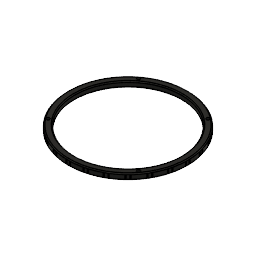
IR Ring v1 (Autodesk Fusion 360 design; units mm, degrees)
Autodesk Fusion 360 part; units mm, degrees
note: some values were not read from the file. Set by a fixed rule: which sketch regions a step uses.
sketch "Sketch1" plane through (0, 0, 0) normal (0, 1, 0) x (1, 0, 0)
  circle A0 centre (0, 0) radius 62 construction
  circle A1 centre (0, 0) radius 65
  circle A2 centre (0, 0) radius 58
  line L0 (0, 0) -> (-49.1879, -37.7432)
  line L1 (0, 0) -> (62, 0) construction
  line L2 (0, 0) -> (-37.7432, 49.1879)
  line L3 (0, 0) -> (0, -65) construction
  line L4 (0, 0) -> (49.1879, -37.7432)
  line L5 (0, 0) -> (37.7432, 49.1879)
  circle A3 centre (-49.1879, -37.7432) radius 1.65
  circle A4 centre (49.1879, -37.7432) radius 1.65
  circle A5 centre (37.7432, 49.1879) radius 1.65
  circle A6 centre (-37.7432, 49.1879) radius 1.65
  line L6 (0, 0) -> (0, 62) construction
  line L7 (3.4, 63.25) -> (-3.4, 63.25)
  line L8 (-3.4, 63.25) -> (-3.4, 60.75)
  line L9 (-3.4, 60.75) -> (3.4, 60.75)
  line L10 (3.4, 60.75) -> (3.4, 63.25)
  line L11 (3.4, 63.25) -> (-3.4, 60.75) construction
  line L12 (-3.4, 63.25) -> (3.4, 60.75) construction
  line L13 (3.6, 60.55) -> (-3.6, 60.55)
  line L14 (-3.6, 60.55) -> (-3.6, 63.45)
  line L15 (-3.6, 63.45) -> (3.6, 63.45)
  line L16 (3.6, 63.45) -> (3.6, 60.55)
  line L17 (3.6, 60.55) -> (-3.6, 63.45) construction
  line L18 (-3.6, 60.55) -> (3.6, 63.45) construction
  line L19 (0, 63.25) -> (1.1, 63.25)
  line L20 (0, 63.25) -> (0.9, 63.25)
  line L21 (0, 63.25) -> (1.7, 63.25)
  circle A7 centre (1.7, 63.25) radius 1.3
  circle A8 centre (1.7, 63.25) radius 1.4
  line L22 (1.1, 63.25) -> (1.1, 64.4033)
  line L23 (0, 63.25) -> (0, 62) construction
  circle A9 centre (-1.7, 63.25) radius 1.4
  circle A10 centre (-1.7, 63.25) radius 1.3
  line L24 (-1.1, 63.45) -> (-1.1, 63.95) construction
  line L25 (-3.6, 63.45) -> (-3.6, 64.9002)
  line L26 (3.6, 63.45) -> (3.6, 64.9002)
  line L27 (-1.1, 63.25) -> (-1.1, 62.0967)
  line L28 (-1.1, 61.9902) -> (-1.1, 61.9851)
  line L29 (1.1, 63.25) -> (1.1, 62.0967)
  line L30 (1.1, 61.9902) -> (1.1, 61.9851)
  line L31 (-1.1, 63.25) -> (-1.1, 64.4033)
  line L32 (-3.6, 60.55) -> (-3.6, 59.55)
  line L33 (-3.6, 59.55) -> (3.6, 59.55)
  line L34 (3.6, 59.55) -> (3.6, 60.55)
  line L35 (3.6, 63.45) -> (3.6, 64.9002)
  line L36 (3.4, 63.25) -> (3.4, 64.911)
  line L37 (-3.4, 63.25) -> (-3.4, 64.911)
  line L38 (1.5, 63.95) -> (-1.5, 63.95)
  line L39 (-3.1, 63.9499) -> (-3.4, 63.95)
  line L40 (-3.4, 63.95) -> (-3.6, 63.95)
  line L41 (3.4, 63.95) -> (3.6, 63.95)
  line L42 (3.1, 63.9499) -> (3.4, 63.95)
  line L43 (-3.6, 63.95) -> (-2.35, 63.95)
  line L44 (3.6, 63.95) -> (2.35, 63.9498)
  line L45 (2.35, 63.9498) -> (2.3499, 64.9575)
  line L46 (-2.35, 63.95) -> (-2.35, 64.9575)
  line L47 (-1.5, 63.95) -> (1.5, 63.95)
  line L48 (-1.5, 63.95) -> (1.5, 63.95)
  line L49 (-1.5, 63.95) -> (-1.5, 64.9827)
  line L50 (1.5, 63.95) -> (1.5, 64.9827)
  point P0 (0, 62)
  point P1 (0, 62)
  point P2 (0, 63.95)
  point P3 (0, 63.95)
  point P4 (0, 63.95)
  point P5 (0, 63.95)
  dimension "d105" = 124
  dimension "d106" = 130
  dimension "d107" = 116
  dimension "d108" = 142.5
  dimension "d109" = 62
  dimension "d110" = 3.3
  dimension "d111" = 3.3
  dimension "d112" = 3.3
  dimension "d113" = 3.3
  dimension "d114" = 6.8
  dimension "d115" = 2.5
  dimension "d116" = 7.2
  dimension "d117" = 2.9
  dimension "d118" = 1.1
  dimension "d119" = 0.9
  dimension "d120" = 1.7
  dimension "d121" = 2.6
  dimension "d122" = 2.8
  dimension "d123" = 0.5
  dimension "d133" = 1
  dimension "d134" = 7.2
  dimension "d136" = 3
  dimension "d142" = 1.6
  dimension "d143" = 1.25
  dimension "d144" = 1.25
  dimension "d145" = 3
  constraint coincident A0.centre A1.centre
  constraint concentric A0 A2
  constraint horizontal L1
  constraint coincident A0 L2.end
  constraint perpendicular L0 L2
  constraint coincident A1 L3.end
  constraint vertical L3
  constraint symmetric A0.centre L3 A1.centre
  constraint symmetric L0.end L3 L4.end
  constraint symmetric L2.end L3 L5.end
  constraint coincident L0.end A3.centre
  constraint coincident L4.end A4.centre
  constraint coincident L5.end A5.centre
  constraint coincident L2.end A6.centre
  constraint coincident A0 P1
  constraint vertical L6
  constraint horizontal L7
  constraint perpendicular L7 L8
  constraint parallel L7 L9
  constraint parallel L8 L10
  constraint coincident L11 P1
  constraint coincident L12 P1
  constraint coincident P1 P0
  constraint horizontal L13
  constraint perpendicular L13 L14
  constraint parallel L13 L15
  constraint parallel L14 L16
  constraint coincident L17 P1
  constraint coincident L18 P1
  constraint midpoint L7 L19.start
  constraint parallel L7 L19
  constraint parallel L19 L20
  constraint parallel L7 L21
  constraint coincident L21.end A7.centre
  constraint concentric A7 A8
  constraint perpendicular L15 L22
  constraint coincident A8 L30.end
  constraint perpendicular L19 L29
  constraint symmetric L19.end L23 L27.start
  constraint symmetric A7 L23 A10
  constraint symmetric A8 L23 A9
  constraint symmetric L30.end L23 L28.end
  constraint coincident L15 L24.start
  constraint perpendicular L15 L24
  constraint coincident A1 L25.end
  constraint perpendicular L15 L25
  constraint coincident A1 L26.end
  constraint perpendicular L15 L26
  constraint coincident A10 L27.end
  constraint coincident A0 L28.start
  constraint collinear L27 L28
  constraint coincident A7 L29.end
  constraint coincident A0 L30.start
  constraint collinear L29 L30
  constraint coincident A7 L22.end
  constraint vertical L31
  constraint coincident A10 L31.end
  constraint perpendicular L13 L32
  constraint perpendicular L32 L33
  constraint coincident A1 L36.end
  constraint perpendicular L7 L36
  constraint coincident A1 L37.end
  constraint perpendicular L15 L37
  constraint midpoint L38 P5
  constraint coincident P5 P4
  constraint coincident L37 L39.end
  constraint coincident L25 L40.end
  constraint perpendicular L25 L40
  constraint symmetric L6 L39.end L41.start
  constraint symmetric L6 L39.start L42.start
  constraint symmetric L6 L40.end L41.end
  constraint perpendicular L25 L43
  constraint parallel L42 L44
  constraint coincident A1 L45.end
  constraint perpendicular L44 L45
  constraint coincident A1 L46.end
  constraint perpendicular L43 L46
  constraint midpoint L47 P5
  constraint midpoint L48 P5
  constraint perpendicular L22 L48
  constraint coincident A1 L49.end
  constraint perpendicular L48 L49
  constraint coincident A1 L50.end
  constraint perpendicular L38 L50
  measures "d105" diameter of A0
  measures "d106" diameter of A1
  measures "d107" diameter of A2
  measures "d108" angle of L0 L1
  measures "d109" distance of A0.centre L0.end
  measures "d110" diameter of A3
  measures "d111" diameter of A4
  measures "d112" diameter of A5
  measures "d113" diameter of A6
  measures "d114" distance of L8.end L9.end
  measures "d115" distance of L7.end L8.end
  measures "d116" distance of L14.end L15.end
  measures "d117" distance of L13.end L14.end
  measures "d118" distance of L19.start L19.end
  measures "d119" distance of L19.start L20.end
  measures "d120" distance of L19.start L21.end
  measures "d121" diameter of A7
  measures "d122" diameter of A8
  measures "d123" distance of L24.start L24.end
  measures "d133" distance of L13.end L32.end
  measures "d134" distance of L32.end L33.end
  measures "d136" distance of L38.end L38.start
  measures "d142" distance of L38.end L39.start
  measures "d143" distance of L40.end L43.end
  measures "d144" distance of L41.end L44.end
  measures "d145" distance of L38.end L38.start
sketch "Sketch2" plane through (0, 0, 0) normal (0, 1, 0) x (1, 0, 0)
  line L0 (0, 0) -> (-43.8406, 43.8406)
  line L1 (0, 0) -> (62, 0) construction
  circle A0 centre (-43.8406, 43.8406) radius 1.65
  line L2 (0, 0) -> (0, 35) construction
  line L3 (0, 0) -> (23, 0) construction
  line L4 (0, 0) -> (0, 50) construction
  circle A1 centre (43.8406, 43.8406) radius 1.65
  circle A2 centre (-43.8406, -43.8406) radius 1.65
  circle A3 centre (43.8406, -43.8406) radius 1.65
  line L5 (-43.8406, 43.8406) -> (-41.7193, 45.9619) construction
  line L6 (-41.7193, 45.9619) -> (-45.9619, 41.7193) construction
  line L7 (-45.9619, 41.7193) -> (-48.7904, 44.5477)
  line L8 (-45.9619, 41.7193) -> (-43.1335, 38.8909)
  line L9 (-43.1335, 38.8909) -> (-38.8909, 43.1335)
  line L10 (-38.8909, 43.1335) -> (-44.5477, 48.7904)
  line L11 (-44.5477, 48.7904) -> (-48.7904, 44.5477)
  line L12 (-43.1335, -38.8909) -> (-48.7904, -44.5477)
  line L13 (-48.7904, -44.5477) -> (-44.5477, -48.7904)
  circle A4 centre (-43.8406, -43.8406) radius 1.65
  line L14 (-41.7193, -45.9619) -> (-44.5477, -48.7904)
  line L15 (-41.7193, -45.9619) -> (-38.8909, -43.1335)
  line L16 (-38.8909, -43.1335) -> (-43.1335, -38.8909)
  line L17 (38.8909, -43.1335) -> (44.5477, -48.7904)
  line L18 (44.5477, -48.7904) -> (48.7904, -44.5477)
  circle A5 centre (43.8406, -43.8406) radius 1.65
  line L19 (45.9619, -41.7193) -> (48.7904, -44.5477)
  line L20 (45.9619, -41.7193) -> (43.1335, -38.8909)
  line L21 (43.1335, -38.8909) -> (38.8909, -43.1335)
  line L22 (43.1335, 38.8909) -> (48.7904, 44.5477)
  line L23 (48.7904, 44.5477) -> (44.5477, 48.7904)
  circle A6 centre (43.8406, 43.8406) radius 1.65
  line L24 (41.7193, 45.9619) -> (44.5477, 48.7904)
  line L25 (41.7193, 45.9619) -> (38.8909, 43.1335)
  line L26 (38.8909, 43.1335) -> (43.1335, 38.8909)
  dimension "d42" = 135
  dimension "d43" = 62
  dimension "d44" = 3.3
  dimension "d45" = 3
  dimension "d46" = 6
  dimension "d48" = 4
  dimension "d49" = 4
  dimension "d50" = 6
  dimension "d51" = 8
  dimension "d53" = 360
  constraint horizontal L1
  constraint coincident L0.start L1.start
  constraint coincident L0.end A0.centre
  constraint perpendicular L1 L2
  constraint coincident L1 L3.end
  constraint symmetric A0 L4 A1
  constraint symmetric L1 A0 A2
  constraint symmetric L1 A1 A3
  constraint perpendicular L0 L5
  constraint parallel L5 L6
  constraint perpendicular L6 L7
  constraint perpendicular L6 L8
  constraint perpendicular L0 L9
  constraint perpendicular L9 L10
  measures "d42" angle of L0 L1
  measures "d43" distance of L0.start L0.end
  measures "d44" diameter of A0
  measures "d45" distance of L0.end L5.end
  measures "d46" distance of L5.end L6.end
  measures "d48" distance of L6.end L7.end
  measures "d49" distance of L6.end L8.end
  measures "d50" distance of L8.end L9.end
  measures "d51" distance of L9.end L10.end
sketch "Sketch3" plane through (0, 0, 0) normal (0, -1, 0) x (1, 0, 0)
  line L0 (43.1335, 38.8909) -> (48.7904, 44.5477)
  line L1 (48.7904, -44.5477) -> (43.1335, -38.8909)
  line L2 (38.8909, -43.1335) -> (44.5477, -48.7904)
  line L3 (-44.5477, -48.7904) -> (-38.8909, -43.1335)
  line L4 (-43.1335, -38.8909) -> (-48.7904, -44.5477)
  line L5 (-48.7904, 44.5477) -> (-43.1335, 38.8909)
  line L6 (-38.8909, 43.1335) -> (-44.5477, 48.7904)
  line L7 (44.5477, 48.7904) -> (38.8909, 43.1335)
  circle A0 centre (-43.8406, -43.8406) radius 1.65
  circle A1 centre (43.8406, -43.8406) radius 1.65
  circle A2 centre (43.8406, 43.8406) radius 1.65
  circle A3 centre (-43.8406, 43.8406) radius 1.65
  circle A4 centre (0, 0) radius 72.5
  circle A5 centre (0, 0) radius 62
  line L8 (0, 0) -> (-50.7874, 35.5617)
  line L9 (0, 0) -> (62, 0) construction
  line L10 (0, 0) -> (50.7874, 35.5617)
  line L11 (0, 0) -> (62, 0) construction
  line L12 (0, 0) -> (-50.7874, -35.5617)
  line L13 (0, 0) -> (50.7874, -35.5617)
  circle A6 centre (-50.7874, 35.5617) radius 1.65
  circle A7 centre (50.7874, 35.5617) radius 1.65
  circle A8 centre (-50.7874, -35.5617) radius 1.65
  circle A9 centre (50.7874, -35.5617) radius 1.65
  line L14 (-50.7874, 35.5617) -> (-46.6917, 32.6939)
  line L15 (-50.7874, 35.5617) -> (-47.9195, 39.6575)
  line L16 (-47.9195, 39.6575) -> (-43.8238, 36.7896)
  line L17 (-46.6917, 32.6939) -> (-43.8238, 36.7896)
  line L18 (-47.9195, 39.6575) -> (-52.0153, 42.5254)
  line L19 (-52.0153, 42.5254) -> (-57.7511, 34.3339)
  line L20 (-57.7511, 34.3339) -> (-49.5595, 28.5981)
  line L21 (-49.5595, 28.5981) -> (-43.8238, 36.7896)
  line L22 (0, 0) -> (0, 16) construction
  line L23 (52.0153, 42.5254) -> (57.7511, 34.3339)
  line L24 (47.9195, 39.6575) -> (52.0153, 42.5254)
  line L25 (47.9195, 39.6575) -> (43.8238, 36.7896)
  line L26 (49.5595, 28.5981) -> (43.8238, 36.7896)
  line L27 (57.7511, 34.3339) -> (49.5595, 28.5981)
  line L28 (-52.0153, -42.5254) -> (-57.7511, -34.3339)
  line L29 (-57.7511, -34.3339) -> (-49.5595, -28.5981)
  line L30 (-49.5595, -28.5981) -> (-43.8238, -36.7896)
  line L31 (-47.9195, -39.6575) -> (-52.0153, -42.5254)
  line L32 (-47.9195, -39.6575) -> (-43.8238, -36.7896)
  line L33 (57.7511, -34.3339) -> (49.5595, -28.5981)
  line L34 (49.5595, -28.5981) -> (43.8238, -36.7896)
  line L35 (47.9195, -39.6575) -> (43.8238, -36.7896)
  line L36 (47.9195, -39.6575) -> (52.0153, -42.5254)
  line L37 (52.0153, -42.5254) -> (57.7511, -34.3339)
  line L38 (44.5477, -48.7904) -> (48.7904, -44.5477)
  line L39 (-44.5477, 48.7904) -> (-48.7904, 44.5477)
  line L40 (48.7904, 44.5477) -> (44.5477, 48.7904)
  line L41 (-48.7904, -44.5477) -> (-44.5477, -48.7904)
  line L42 (38.8909, 43.1335) -> (43.1335, 38.8909)
  line L43 (-38.8909, -43.1335) -> (-43.1335, -38.8909)
  line L44 (43.1335, -38.8909) -> (38.8909, -43.1335)
  line L45 (-43.1335, 38.8909) -> (-38.8909, 43.1335)
  dimension "d58" = 145
  dimension "d59" = 35
  dimension "d60" = 3.3
  dimension "d61" = 3.3
  dimension "d62" = 3.3
  dimension "d63" = 3.3
  dimension "d64" = 5
  dimension "d65" = 5
  dimension "d66" = 5
  dimension "d67" = 5
  dimension "d69" = 10
  dimension "d70" = 10
  constraint concentric A4 A5
  constraint coincident A3.centre A5
  constraint horizontal L9
  constraint coincident A4.centre A5.centre
  constraint horizontal L11
  constraint coincident A5 L10.end
  constraint coincident A5 L12.end
  constraint parallel L10 L12
  constraint coincident A5 L13.end
  constraint parallel L8 L13
  constraint coincident L8.end A6.centre
  constraint coincident L10.end A7.centre
  constraint coincident L12.end A8.centre
  constraint coincident L13.end A9.centre
  constraint parallel L8 L14
  constraint perpendicular L8 L15
  constraint perpendicular L15 L16
  constraint perpendicular L15 L18
  constraint perpendicular L18 L19
  constraint perpendicular L19 L20
  constraint vertical L22
  constraint symmetric L15.end L22 L24.start
  constraint symmetric L16.end L22 L25.end
  constraint symmetric L18.end L22 L23.start
  constraint symmetric L19.end L22 L23.end
  constraint symmetric L20.end L22 L26.start
  constraint symmetric L11 L15.end L31.start
  constraint symmetric L11 L16.end L30.end
  constraint symmetric L11 L18.end L28.start
  constraint symmetric L11 L19.end L28.end
  constraint symmetric L11 L20.end L29.end
  constraint symmetric L11 L23.start L36.end
  constraint symmetric L11 L23.end L33.start
  constraint symmetric L11 L24.start L35.start
  constraint symmetric L11 L25.end L34.end
  constraint symmetric L11 L26.start L33.end
  measures "d58" angle of L8 L9
  measures "d59" angle of L10 L11
  measures "d60" diameter of A6
  measures "d61" diameter of A7
  measures "d62" diameter of A8
  measures "d63" diameter of A9
  measures "d64" distance of L8.end L14.end
  measures "d65" distance of L8.end L15.end
  measures "d66" distance of L15.end L16.end
  measures "d67" distance of L15.end L18.end
  measures "d69" distance of L18.end L19.end
  measures "d70" distance of L19.end L20.end
sketch "Sketch4" plane through (0, 5, 0) normal (0, 1, 0) x (-1, 0, 0)
  circle A0 centre (-50.7874, 35.5617) radius 1.65
  circle A1 centre (-50.7874, -35.5617) radius 1.65
  circle A2 centre (50.7874, -35.5617) radius 1.65
  circle A3 centre (50.7874, 35.5617) radius 1.65
  line L0 (50.7874, 35.5617) -> (53.7874, 35.5617)
  line L1 (50.7874, 35.5617) -> (52.2874, 38.1598)
  line L2 (50.7874, 35.5617) -> (49.2874, 38.1598)
  line L3 (50.7874, 35.5617) -> (47.7874, 35.5617)
  line L4 (50.7874, 35.5617) -> (49.2874, 32.9637)
  line L5 (50.7874, 35.5617) -> (52.2874, 32.9637)
  line L6 (49.2874, 38.1598) -> (52.2874, 38.1598)
  line L7 (52.2874, 38.1598) -> (53.7874, 35.5617)
  line L8 (53.7874, 35.5617) -> (52.2874, 32.9637)
  line L9 (52.2874, 32.9637) -> (49.2874, 32.9637)
  line L10 (49.2874, 32.9637) -> (47.7874, 35.5617)
  line L11 (47.7874, 35.5617) -> (49.2874, 38.1598)
  line L12 (0, 0) -> (0, 25) construction
  line L13 (0, 0) -> (25, 0) construction
  line L14 (-49.2874, 38.1598) -> (-52.2874, 38.1598)
  line L15 (-47.7874, 35.5617) -> (-49.2874, 38.1598)
  line L16 (-49.2874, 32.9637) -> (-47.7874, 35.5617)
  line L17 (-52.2874, 32.9637) -> (-49.2874, 32.9637)
  line L18 (-53.7874, 35.5617) -> (-52.2874, 32.9637)
  line L19 (-52.2874, 38.1598) -> (-53.7874, 35.5617)
  line L20 (-49.2874, -38.1598) -> (-52.2874, -38.1598)
  line L21 (-52.2874, -38.1598) -> (-53.7874, -35.5617)
  line L22 (-53.7874, -35.5617) -> (-52.2874, -32.9637)
  line L23 (-52.2874, -32.9637) -> (-49.2874, -32.9637)
  line L24 (-49.2874, -32.9637) -> (-47.7874, -35.5617)
  line L25 (-47.7874, -35.5617) -> (-49.2874, -38.1598)
  line L26 (49.2874, -38.1598) -> (52.2874, -38.1598)
  line L27 (47.7874, -35.5617) -> (49.2874, -38.1598)
  line L28 (49.2874, -32.9637) -> (47.7874, -35.5617)
  line L29 (52.2874, -32.9637) -> (49.2874, -32.9637)
  line L30 (53.7874, -35.5617) -> (52.2874, -32.9637)
  line L31 (52.2874, -38.1598) -> (53.7874, -35.5617)
  circle A4 centre (-43.8406, 43.8406) radius 1.65
  line L32 (-48.7904, 44.5477) -> (-43.1335, 38.8909)
  line L33 (-43.1335, 38.8909) -> (-38.8909, 43.1335)
  line L34 (-38.8909, 43.1335) -> (-44.5477, 48.7904)
  line L35 (-44.5477, 48.7904) -> (-48.7904, 44.5477)
  circle A5 centre (43.8406, -43.8406) radius 1.65
  line L36 (48.7904, -44.5477) -> (43.1335, -38.8909)
  line L37 (43.1335, -38.8909) -> (38.8909, -43.1335)
  line L38 (38.8909, -43.1335) -> (44.5477, -48.7904)
  line L39 (44.5477, -48.7904) -> (48.7904, -44.5477)
  circle A6 centre (43.8406, 43.8406) radius 1.65
  line L40 (44.5477, 48.7904) -> (38.8909, 43.1335)
  line L41 (38.8909, 43.1335) -> (43.1335, 38.8909)
  line L42 (43.1335, 38.8909) -> (48.7904, 44.5477)
  line L43 (48.7904, 44.5477) -> (44.5477, 48.7904)
  circle A7 centre (-43.8406, -43.8406) radius 1.65
  line L44 (-44.5477, -48.7904) -> (-38.8909, -43.1335)
  line L45 (-38.8909, -43.1335) -> (-43.1335, -38.8909)
  line L46 (-43.1335, -38.8909) -> (-48.7904, -44.5477)
  line L47 (-48.7904, -44.5477) -> (-44.5477, -48.7904)
  dimension "d75" = 3
  dimension "d77" = 360
  constraint coincident A3.centre L0.start
  constraint horizontal L0
  constraint coincident L12.start L13.start
  constraint vertical L12
  constraint perpendicular L12 L13
  constraint symmetric L0.end L12 L18.start
  constraint symmetric L1.end L12 L14.end
  constraint symmetric L2.end L12 L14.start
  constraint symmetric L3.end L12 L15.start
  constraint symmetric L4.end L12 L16.start
  constraint symmetric L5.end L12 L17.start
  constraint symmetric L0.end L13 L30.start
  constraint symmetric L1.end L13 L26.end
  constraint symmetric L2.end L13 L26.start
  constraint symmetric L3.end L13 L27.start
  constraint symmetric L4.end L13 L28.start
  constraint symmetric L5.end L13 L29.start
  constraint symmetric L13 L14.start L20.start
  constraint symmetric L13 L14.end L20.end
  constraint symmetric L13 L15.start L24.end
  constraint symmetric L13 L16.start L23.end
  constraint symmetric L13 L17.start L22.end
  constraint symmetric L13 L18.start L21.end
  measures "d75" distance of A3.centre L0.end
sketch "Sketch5" plane through (0, 5, 0) normal (0, 1, 0) x (-1, 0, 0)
  circle A0 centre (-43.8406, -43.8406) radius 1.65
  circle A1 centre (43.8406, 43.8406) radius 1.65
  circle A2 centre (-43.8406, 43.8406) radius 1.65
  circle A3 centre (43.8406, -43.8406) radius 1.65
  line L0 (-43.1335, -38.8909) -> (-48.7904, -44.5477)
  line L1 (-48.7904, 44.5477) -> (-43.1335, 38.8909)
  line L2 (-38.8909, 43.1335) -> (-44.5477, 48.7904)
  line L3 (44.5477, 48.7904) -> (38.8909, 43.1335)
  line L4 (43.1335, 38.8909) -> (48.7904, 44.5477)
  line L5 (48.7904, -44.5477) -> (43.1335, -38.8909)
  line L6 (38.8909, -43.1335) -> (44.5477, -48.7904)
  line L7 (-44.5477, -48.7904) -> (-38.8909, -43.1335)
  circle A4 centre (0, 0) radius 68.75
  line L8 (0, 0) -> (0, -68.75)
  line L9 (0, 0) -> (17.7938, -66.4074)
  line L10 (0, 0) -> (34.375, -59.5392)
  line L11 (0, 0) -> (48.6136, -48.6136)
  line L12 (0, 0) -> (59.5392, -34.375)
  line L13 (0, 0) -> (66.4074, -17.7938)
  line L14 (0, 0) -> (68.75, 0)
  line L15 (0, 0) -> (66.4074, 17.7938)
  line L16 (0, 0) -> (59.5392, 34.375)
  line L17 (0, 0) -> (48.6136, 48.6136)
  line L18 (0, 0) -> (34.375, 59.5392)
  line L19 (0, 0) -> (17.7938, 66.4074)
  line L20 (0, 0) -> (0, 68.75)
  line L21 (0, 0) -> (-17.7938, 66.4074)
  line L22 (0, 0) -> (-34.375, 59.5392)
  line L23 (0, 0) -> (-48.6136, 48.6136)
  line L24 (0, 0) -> (-59.5392, 34.375)
  line L25 (0, 0) -> (-66.4074, 17.7938)
  line L26 (0, 0) -> (-68.75, 0)
  line L27 (0, 0) -> (-66.4074, -17.7938)
  line L28 (0, 0) -> (-59.5392, -34.375)
  line L29 (0, 0) -> (-48.6136, -48.6136)
  line L30 (0, 0) -> (-34.375, -59.5392)
  line L31 (0, 0) -> (-17.7938, -66.4074)
  line L32 (34.375, -59.5392) -> (17.7938, -66.4074)
  line L33 (26.0844, -62.9733) -> (26.3095, -63.5167)
  circle A5 centre (26.3095, -63.5167) radius 1.65
  line L34 (26.3095, -63.5167) -> (23.5378, -64.6648)
  line L35 (26.3095, -63.5167) -> (25.9179, -66.4911)
  line L36 (26.3095, -63.5167) -> (28.6895, -65.343)
  line L37 (26.3095, -63.5167) -> (29.0811, -62.3687)
  line L38 (26.3095, -63.5167) -> (26.7011, -60.5424)
  line L39 (26.3095, -63.5167) -> (23.9294, -61.6904)
  line L40 (29.0811, -62.3687) -> (28.6895, -65.343)
  line L41 (29.0811, -62.3687) -> (26.7011, -60.5424)
  line L42 (26.7011, -60.5424) -> (23.9294, -61.6904)
  line L43 (23.5378, -64.6648) -> (23.9294, -61.6904)
  line L44 (23.5378, -64.6648) -> (25.9179, -66.4911)
  line L45 (25.9179, -66.4911) -> (28.6895, -65.343)
  line L46 (62.3687, -29.0811) -> (65.343, -28.6895)
  line L47 (65.343, -28.6895) -> (66.4911, -25.9179)
  line L48 (64.6648, -23.5378) -> (66.4911, -25.9179)
  line L49 (64.6648, -23.5378) -> (61.6904, -23.9294)
  line L50 (61.6904, -23.9294) -> (60.5424, -26.7011)
  line L51 (62.3687, -29.0811) -> (60.5424, -26.7011)
  circle A6 centre (63.5167, -26.3095) radius 1.65
  line L52 (64.6648, 23.5378) -> (66.4911, 25.9179)
  line L53 (66.4911, 25.9179) -> (65.343, 28.6895)
  line L54 (62.3687, 29.0811) -> (65.343, 28.6895)
  line L55 (62.3687, 29.0811) -> (60.5424, 26.7011)
  line L56 (60.5424, 26.7011) -> (61.6904, 23.9294)
  line L57 (64.6648, 23.5378) -> (61.6904, 23.9294)
  circle A7 centre (63.5167, 26.3095) radius 1.65
  line L58 (29.0811, 62.3687) -> (28.6895, 65.343)
  line L59 (28.6895, 65.343) -> (25.9179, 66.4911)
  line L60 (23.5378, 64.6648) -> (25.9179, 66.4911)
  line L61 (23.5378, 64.6648) -> (23.9294, 61.6904)
  line L62 (23.9294, 61.6904) -> (26.7011, 60.5424)
  line L63 (29.0811, 62.3687) -> (26.7011, 60.5424)
  circle A8 centre (26.3095, 63.5167) radius 1.65
  line L64 (-23.5378, 64.6648) -> (-25.9179, 66.4911)
  line L65 (-25.9179, 66.4911) -> (-28.6895, 65.343)
  line L66 (-29.0811, 62.3687) -> (-28.6895, 65.343)
  line L67 (-29.0811, 62.3687) -> (-26.7011, 60.5424)
  line L68 (-26.7011, 60.5424) -> (-23.9294, 61.6904)
  line L69 (-23.5378, 64.6648) -> (-23.9294, 61.6904)
  circle A9 centre (-26.3095, 63.5167) radius 1.65
  line L70 (-62.3687, 29.0811) -> (-65.343, 28.6895)
  line L71 (-65.343, 28.6895) -> (-66.4911, 25.9179)
  line L72 (-64.6648, 23.5378) -> (-66.4911, 25.9179)
  line L73 (-64.6648, 23.5378) -> (-61.6904, 23.9294)
  line L74 (-61.6904, 23.9294) -> (-60.5424, 26.7011)
  line L75 (-62.3687, 29.0811) -> (-60.5424, 26.7011)
  circle A10 centre (-63.5167, 26.3095) radius 1.65
  line L76 (-64.6648, -23.5378) -> (-66.4911, -25.9179)
  line L77 (-66.4911, -25.9179) -> (-65.343, -28.6895)
  line L78 (-62.3687, -29.0811) -> (-65.343, -28.6895)
  line L79 (-62.3687, -29.0811) -> (-60.5424, -26.7011)
  line L80 (-60.5424, -26.7011) -> (-61.6904, -23.9294)
  line L81 (-64.6648, -23.5378) -> (-61.6904, -23.9294)
  circle A11 centre (-63.5167, -26.3095) radius 1.65
  line L82 (-29.0811, -62.3687) -> (-28.6895, -65.343)
  line L83 (-28.6895, -65.343) -> (-25.9179, -66.4911)
  line L84 (-23.5378, -64.6648) -> (-25.9179, -66.4911)
  line L85 (-23.5378, -64.6648) -> (-23.9294, -61.6904)
  line L86 (-23.9294, -61.6904) -> (-26.7011, -60.5424)
  line L87 (-29.0811, -62.3687) -> (-26.7011, -60.5424)
  circle A12 centre (-26.3095, -63.5167) radius 1.65
  line L88 (38.8909, 43.1335) -> (43.1335, 38.8909)
  line L89 (48.7904, 44.5477) -> (44.5477, 48.7904)
  line L90 (-43.1335, 38.8909) -> (-38.8909, 43.1335)
  line L91 (-44.5477, 48.7904) -> (-48.7904, 44.5477)
  line L92 (-38.8909, -43.1335) -> (-43.1335, -38.8909)
  line L93 (-48.7904, -44.5477) -> (-44.5477, -48.7904)
  line L94 (43.1335, -38.8909) -> (38.8909, -43.1335)
  line L95 (44.5477, -48.7904) -> (48.7904, -44.5477)
  dimension "d88" = 137.5
  dimension "d90" = 360
  dimension "d91" = 3.3
  dimension "d92" = 3
  dimension "d94" = 360
  dimension "d96" = 360
  constraint coincident A4.centre L8.start
  constraint coincident A4 L8.end
  constraint vertical L8
  constraint midpoint L32 L33.start
  constraint coincident A4 L33.end
  constraint perpendicular L32 L33
  constraint coincident L33.end A5.centre
  constraint perpendicular L33 L34
  measures "d88" diameter of A4
  measures "d91" diameter of A5
  measures "d92" distance of L33.end L34.end
extrude "Extrude13" add sketch "Sketch1" along normal blind 6
sketch "Sketch6" plane through (0, 0, 0) normal (0, -1, 0) x (1, 0, 0)
  circle A0 centre (0, 0) radius 58
  circle A1 centre (0, 0) radius 65
  circle A2 centre (0, 0) radius 64
  circle A3 centre (-49.1879, 37.7432) radius 1.65
  circle A4 centre (0, 0) radius 58
  circle A5 centre (49.1879, 37.7432) radius 1.65
  circle A6 centre (-37.7432, -49.1879) radius 1.65
  circle A7 centre (37.7432, -49.1879) radius 1.65
  circle A8 centre (0, 0) radius 65
  line L0 (0, 0) -> (0, -64) construction
  line L1 (0, -64) -> (0, -59.5499) construction
  line L2 (0, -59.5499) -> (3.6, -59.5499)
  line L3 (3.6, -59.5499) -> (3.6, -63.8987)
  line L4 (0, -59.5499) -> (-3.6, -59.5499)
  line L5 (-3.6, -59.5499) -> (-3.6, -63.8987)
  dimension "d137" = 130
  dimension "d152" = 3.6
  dimension "d153" = 3.6
  constraint concentric A0 A1
  constraint concentric A0 A2
  constraint coincident A0.centre A1.centre
  constraint coincident A2 L0.end
  constraint vertical L0
  constraint coincident L0 L1.end
  constraint perpendicular L0 L2
  constraint coincident A2 L3.end
  constraint perpendicular L2 L3
  constraint perpendicular L1 L4
  constraint coincident A2 L5.end
  constraint perpendicular L4 L5
  measures "d137" diameter of A1
  measures "d152" distance of L1.end L2.end
  measures "d153" distance of L1.end L4.end
extrude "Extrude16" cut sketch "Sketch1" along normal blind 4.5 contours L15 L26 L35 L36 L41 L44 | L15 L25 L37 L40 L43 | A1 A8 L45 L50 | L15 A8 L36 L42 L44 | L8 L9 L10 L13 L14 L15 L16 L36 L37 | A1 A9 L46 L49 | L15 A9 L37 L39 L43 | A7 A8 L45 L50 | L7 L15 A8 L36 | L13 L32 L33 L34 | A9 A10 L46 L49 | L7 L15 A9 L37 | L15 A7 A8 L44 | L15 A7 L22 L38 L44 L45 L47 L48 L50 | L7 L15 A7 A8 | L7 L8 L9 L10 L19 L20 L21 A8 A9 | L15 A9 A10 L43 | L15 A10 L31 L38 L43 L46 L47 L48 L49 | L7 L15 A9 A10 | L15 A7 A8 L38 L47 L48 | L15 A8 A9 L38 L47 L48 | L7 L15 L21 A7 L22 | L7 L19 L20 L21 A7 A8 | L15 A9 A10 L38 L47 L48 | L7 L15 A10 L31 | L7 A9 A10 | L7 L15 L19 L20 L21 A8 A9 | L7 L15 L19 L20 L21 A7 A8 | L15 A7 L22 L38 L47 L48 | L7 L15 L19 L20 L21 A7 L22 | L7 L21 A7 L29 | L7 L15 A9 A10 | L15 A10 L31 L38 L47 L48 | L7 L15 A10 L31 | L7 A10 L27 | L7 L19 L20 L21 A7 L29 | L7 A10 L27
pattern_circular "C-Pattern4" count 24 over 360 about axis through (0, 1.75, 0) along (0, 1, 0) of "Extrude16"
extrude "Extrude17" add sketch "Sketch6" against normal blind 1 contours A1 A8 | A2 L2 L3 L4 L5 | A2 L2 L3 L4 L5
extrude "Extrude18" cut sketch "Sketch6" against normal blind 1 contours A2 L2 L3 L4 L5 picked at (-1.6002, -61.0295)
pattern_circular "C-Pattern5" count 24 over 360 about axis through (0, 1.75, 0) along (0, 1, 0) of "Extrude18"
fillet "Fillet7" radius 1 1 edges at (-60.6013, 6, 23.505)
fillet "Fillet8" radius 0.5 1 edges at (-60.6013, 0, 23.505)
fillet "Fillet9" radius 0.35 8 edges at (-34.2619, 4.5, 54.6435) (-33.5322, 4.5, 55.0795) (-30.1917, 4.5, 56.9936) (-30.9341, 4.5, 56.5795) (-34.2637, 1, 54.6466) (-33.5403, 1, 55.0935) (-30.1934, 1, 56.9965) (-30.9422, 1, 56.5935)
fillet "Fillet10" radius 1 2 edges at (-54.075, 6, -20.9737) (-54.075, 0, -20.9737)
equation "d59 = 180 deg - 145 deg"
equation "d105 = ( 62 * 2 ) * 1 mm"
equation "d107 = ( 58 * 2 ) * 1 mm"
